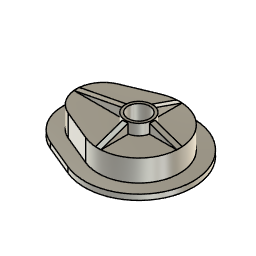
18 (Autodesk Fusion 360 design; units mm, degrees)
Autodesk Fusion 360 part; units mm, degrees
sketch "草图1" plane through (0, 0, 0) normal (0, 0, 1) x (1, 0, 0)
  line L0 (-140, 0) -> (100, 0) construction
  circle A0 centre (0, 0) radius 8
  circle A1 centre (0, 0) radius 10
  line L1 (-37.5385, 27.6923) -> (-15.3846, 36.9231)
  line L2 (-15.3846, -36.9231) -> (-37.5385, -27.6923)
  arc A2 (-37.5385, 27.6923) -> (-37.5385, -27.6923) centre (-26, 0) ccw
  line L3 (-33.6923, 18.4615) -> (-11.5385, 27.6923)
  line L4 (-11.5385, -27.6923) -> (-33.6923, -18.4615)
  arc A3 (-33.6923, 18.4615) -> (-33.6923, -18.4615) centre (-26, 0) ccw
  arc A4 (-11.5385, -27.6923) -> (-11.5385, 27.6923) centre (0, 0) ccw
  arc A5 (-15.3846, -36.9231) -> (-15.3846, 36.9231) centre (0, 0) ccw
  dimension "d1" = 20
  dimension "d2" = 16
  dimension "d3" = 80
  dimension "d4" = 60
  dimension "d5" = 60
  dimension "d6" = 40
  dimension "d7" = 26
  constraint horizontal L0
  constraint coincident A0.centre A1.centre
  constraint concentric A0 A1
  constraint concentric A0 A5
  constraint concentric A0 A4
  constraint coincident L0 A2.centre
  constraint concentric A2 A3
  constraint tangent L1 A5
  constraint tangent L2 A5
  constraint tangent L2 A2
  constraint tangent L1 A2
  constraint tangent L3 A4
  constraint tangent L3 A3
  constraint tangent L4 A3
  constraint tangent L4 A4
  measures "d1" diameter of A1
  measures "d2" diameter of A0
  measures "d3" diameter of A5
  measures "d4" diameter of A4
  measures "d5" diameter of A2
  measures "d6" diameter of A3
  measures "d7" distance of A0.centre A2.centre
extrude "拉伸1" add sketch "草图1" against normal blind 4 contours A1 | L1 L2 A2 A5 | L3 L4 A3 A4 makes body 1
extrude "拉伸2" add sketch "草图1" along normal blind 16 contours A1 | L3 L4 A3 A4 bodies 1
extrude "拉伸3" add sketch "草图1" along normal blind 24 contours A1 bodies 1
sketch "草图2" plane through (0, 0, -4) normal (0, 0, -1) x (1, 0, 0)
  circle A0 centre (0, 0) radius 8
  arc A1 (-37.5385, 27.6923) -> (-37.5385, -27.6923) centre (-26, 0) ccw
  line L0 (-37.5385, -27.6923) -> (-15.3846, -36.9231)
  arc A2 (-15.3846, -36.9231) -> (-15.3846, 36.9231) centre (0, 0) ccw
  line L1 (-15.3846, 36.9231) -> (-37.5385, 27.6923)
  circle A3 centre (0, 0) radius 8
  circle A4 centre (0, 0) radius 10
  line L2 (-31.7692, 13.8462) -> (-9.6154, 23.0769)
  line L3 (-9.6154, -23.0769) -> (-31.7692, -13.8462)
  arc A5 (-31.7692, 13.8462) -> (-31.7692, -13.8462) centre (-26, 0) ccw
  arc A6 (-9.6154, -23.0769) -> (-9.6154, 23.0769) centre (0, 0) ccw
  line L4 (-66, 0) -> (45, 0) construction
  dimension "d14" = 50
  dimension "d15" = 30
  dimension "d16" = 20
  dimension "d17" = 16
  dimension "d18" = 26
  constraint coincident A0.centre A2.centre
  constraint tangent L2 A6
  constraint tangent L2 A5
  constraint tangent L3 A5
  constraint tangent L3 A6
  constraint horizontal L4
  constraint collinear A1.centre L4.start L4.end
  measures "d14" diameter of A6
  measures "d15" diameter of A5
  measures "d16" diameter of A4
  measures "d17" diameter of A3
  measures "d18" distance of A0.centre A1.centre
extrude "拉伸4" cut sketch "草图2" against normal blind 16 contours L2 L3 A5 A6 bodies 1
extrude "拉伸5" cut 1 faces at (9.2663, 0.8943, -4) along direction (0, 0, 1) blind 11 on bodies 1 bodies 1
sketch "草图3" plane through (0, 0, 0) normal (0, 1, 0) x (1, 0, 0)
  line L0 (-10, -24) -> (10, -24)
  line L1 (10, -24) -> (10, -23)
  line L2 (10, -23) -> (-10, -23)
  line L3 (-10, -23) -> (-10, -24)
  line L4 (-10, -23) -> (-46, -16)
  line L5 (-46, -16) -> (30, -16)
  line L6 (30, -16) -> (10, -23)
  line L7 (-10, -23) -> (-10, -16)
  line L8 (10, -23) -> (10, -16)
  dimension "d23" = 1
  dimension "d24" = 20
  constraint horizontal L0
  constraint perpendicular L0 L1
  constraint perpendicular L1 L2
  constraint perpendicular L0 L3
  constraint perpendicular L1 L5
  constraint coincident L5 L7.end
  constraint perpendicular L5 L7
  constraint coincident L5 L8.end
  constraint perpendicular L5 L8
  measures "d23" distance of L0.end L1.end
  measures "d24" distance of L0.start L0.end
extrude "拉伸6" add sketch "草图3" along normal mid plane 4 separate body contours L4 L5 L7 | L5 L6 L8 makes body 2 at (16.6667, 0.6667, 20.6667) makes body 3 at (-34, 0.6667, 18.3333)
sketch "草图4" plane through (0, 0, 0) normal (1, 0, 0) x (0, 1, 0)
  line L0 (-10, 24) -> (10, 24)
  line L1 (10, 24) -> (10, 23)
  line L2 (10, 23) -> (30, 16)
  line L3 (30, 16) -> (-30, 16)
  line L4 (-30, 16) -> (-10, 23)
  line L5 (-10, 23) -> (-10, 24)
  line L6 (-10, 23) -> (-10, 16)
  line L7 (10, 23) -> (10, 16)
  constraint horizontal L0
  constraint perpendicular L0 L1
  constraint perpendicular L1 L3
  constraint perpendicular L0 L5
  constraint coincident L3 L6.end
  constraint perpendicular L3 L6
  constraint coincident L3 L7.end
  constraint perpendicular L3 L7
extrude "拉伸7" add sketch "草图4" along normal mid plane 4 separate body contours L3 L4 L6 | L2 L3 L7 makes body 4 at (0.6667, 23.3333, 18.3333) makes body 5 at (0.6667, -16.6667, 20.6667)
extrude "拉伸8" cut 1 faces at (-17.8311, -17.2623, 16) along direction (0, 0, 1) blind 18 keep common part on bodies 1 bodies 2 3 4 5
